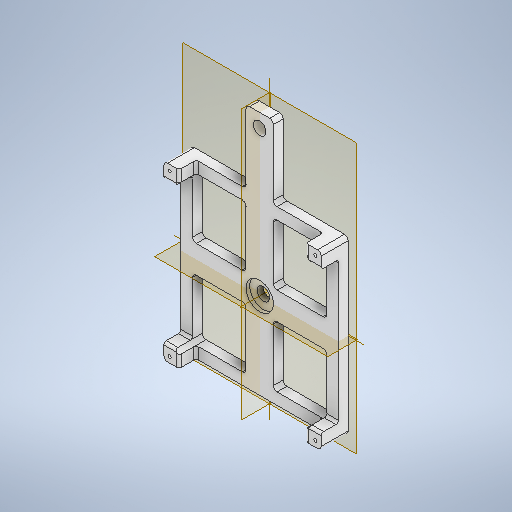
# Autodesk Inventor part: box-mount
Saved by Autodesk Inventor 2025.2 (Build 292293000, 293)
## iProperties
Created: 2025-04-08
Part Number: box-mount
Material: ABS Plastic
Document SubType Name: Modeling
Designer: yehorderehus
Density: 1.06 g/cm^3
Appearance: Smooth - White
Author: yehorderehus
Autodesk Inventor part; units mm, degrees
sketch "Sketch1" plane through (0, 0, 0) normal (0, 0, 1) x (1, 0, 0)
  line L0 (64.25, -70.25) -> (-64.25, -70.25)
  line L1 (-64.25, -70.25) -> (-64.25, 70.25)
  line L2 (-64.25, 70.25) -> (64.25, 70.25)
  line L3 (64.25, 70.25) -> (64.25, -70.25)
  circle A0 centre (0, 0) radius 5.2
  circle A1 centre (-59.5, -65.5) radius 1.25
  circle A2 centre (59.5, -65.5) radius 1.25
  circle A3 centre (59.5, 65.5) radius 1.25
  circle A4 centre (-59.5, 65.5) radius 1.25
  line L4 (-11.2, 70.25) -> (11.2, 70.25)
  line L5 (11.2, 70.25) -> (11.2, 129.75)
  line L6 (11.2, 129.75) -> (-11.2, 129.75)
  line L7 (-11.2, 129.75) -> (-11.2, 70.25)
  line L8 (0, 169.75) -> (0, -110.25) projected
  circle A5 centre (0, 118.55) radius 5.2
  line L9 (-54.75, 60.75) -> (-11.2, 60.75)
  line L10 (-11.2, 60.75) -> (-11.2, 11.2)
  line L11 (-11.2, 11.2) -> (-54.75, 11.2)
  line L12 (-54.75, 11.2) -> (-54.75, 60.75)
  line L13 (11.2, 11.2) -> (54.75, 11.2)
  line L14 (54.75, 11.2) -> (54.75, 60.75)
  line L15 (54.75, 60.75) -> (11.2, 60.75)
  line L16 (11.2, 60.75) -> (11.2, 11.2)
  line L17 (-11.2, -11.2) -> (-54.75, -11.2)
  line L18 (-54.75, -11.2) -> (-54.75, -60.75)
  line L19 (-54.75, -60.75) -> (-11.2, -60.75)
  line L20 (-11.2, -60.75) -> (-11.2, -11.2)
  line L21 (11.2, -11.2) -> (54.75, -11.2)
  line L22 (54.75, -11.2) -> (54.75, -60.75)
  line L23 (54.75, -60.75) -> (11.2, -60.75)
  line L24 (11.2, -60.75) -> (11.2, -11.2)
  line L25 (-89.95, 0) -> (89.95, 0) projected
  point P0 (11.2, 70.25)
  dimension "d0" = 10.4
  dimension "d12" = 119
  dimension "d14" = 131
  dimension "d44" = 3.5
  dimension "d45" = 3.5
  dimension "d46" = 3.5
  dimension "d47" = 3.5
  dimension "d48" = 3.5
  dimension "d49" = 3.5
  dimension "d50" = 6
  dimension "d51" = 6
  dimension "d52" = 3.5
  dimension "d53" = 65.5
  dimension "d54" = 2.5
  dimension "d55" = 59.5
  dimension "d56" = 6
  dimension "d57" = 3.5
  dimension "d58" = 6
  dimension "d60" = 6
  dimension "d62" = 200
  dimension "d63" = 118.55
  constraints: 48 end point, 12 equal length, 8 vertical alignment, 7 coincident, 6 centre point, 6 horizontal, 6 perpendicular, 4 equal radius, 4 horizontal alignment, 4 point on line
  measures "d0" diameter of A0
  measures "d12" distance of A1.centre A2.centre
  measures "d14" distance of A1.centre A4.centre
  measures "d44" distance edge to line of A1 L1
  measures "d45" distance edge to line of A1 L0
  measures "d46" distance edge to line of A4 L2
  measures "d47" distance edge to line of A2 L3
  measures "d48" distance edge to line of A1 L18
  measures "d49" distance edge to line of A2 L22
  measures "d50" distance edge to line of A0 L20
  measures "d51" distance edge to line of A0 L24
  measures "d52" distance edge to line of A1 L19
  measures "d53" distance from line of A1.centre L25
  measures "d54" diameter of A1
  measures "d55" distance from line of A1.centre L8
  measures "d56" distance edge to line of A0 L17
  measures "d57" distance edge to line of A4 L9
  measures "d58" distance edge to line of A0 L11
  measures "d60" distance edge to line of A5 L6
  measures "d62" distance between parallel lines of L0 L6
  measures "d63" distance of A0.centre A5.centre
extrude "Extrusion1" add sketch "Sketch1" along normal blind 8 contours L0 L8 A0 L25 L3 | L0 L1 L25 A0 L8 | L25 A0 L8 L2 L3 | L8 L25 A0 | A0 L25 L8 | L25 L8 A0 | L1 L2 L8 A0 L25 | A0 L8 L25 | L2 L8 A5 L6 L5 | L2 L7 L6 L8 A5 | A5 L8 | L8 A5 | A1 | A2 | A3 | A4
fillet "Fillet1" radius 3 24 edges at (64.25, 70.25, 4) (-64.25, 70.25, 4) (64.25, -70.25, 4) (-64.25, -70.25, 4) (11.2, 129.75, 4) (-11.2, 129.75, 4) (11.2, 70.25, 4) (-11.2, 70.25, 4) (-54.75, 60.75, 4) (-11.2, 60.75, 4) (-11.2, 11.2, 4) (-54.75, 11.2, 4) (11.2, 60.75, 4) (54.75, 60.75, 4) (11.2, 11.2, 4) (54.75, 11.2, 4) (-11.2, -11.2, 4) (-54.75, -11.2, 4) (-11.2, -60.75, 4) (-54.75, -60.75, 4) (11.2, -60.75, 4) (11.2, -11.2, 4) (54.75, -11.2, 4) (54.75, -60.75, 4)
hole "Hole1" at (59.5, 65.5, 0) at (-59.5, 65.5, 0) at (-59.5, -65.5, 0) at (59.5, -65.5, 0) direction (0, 0, 1) diameter 2.5 depth 8 counterbore diameter 6.4 counterbore depth 2
sketch "Sketch2" plane through (0, 0, 8) normal (0, 0, 1) x (1, 0, 0)
  line L0 (-89.95, 0) -> (89.95, 0) projected
  line L1 (0, 169.75) -> (0, -110.25) projected
  point P0 (0, 0)
  point P1 (0, 0)
  point P2 (0, 118.55)
  dimension "d71" = 118.55
  constraints: 1 coincident, 1 point on line
  measures "d71" distance from line of L0 point (0, 118.55)
hole "Hole2" at (0, 0, 8) direction (0, 0, -1) diameter 10.4 depth 8 counterbore diameter 22.4 counterbore depth 3
hole "Hole3" at (0, 118.55, 8) direction (0, 0, -1) diameter 10.4 depth 8
sketch "Sketch3" plane through (0, 0, 8) normal (0, 0, 1) x (1, 0, 0)
  circle A0 centre (-59.5, 65.5) radius 1.25 projected
  circle A1 centre (59.5, 65.5) radius 1.25 projected
  circle A2 centre (59.5, -65.5) radius 1.25 projected
  circle A3 centre (-59.5, -65.5) radius 1.25 projected
  arc A4 (-54.75, -57.75) -> (-51.75, -60.75) centre (-51.75, -57.75) ccw projected
  arc A5 (-51.75, 60.75) -> (-54.75, 57.75) centre (-51.75, 57.75) ccw projected
  arc A6 (54.75, 57.75) -> (51.75, 60.75) centre (51.75, 57.75) ccw projected
  arc A7 (64.25, 67.25) -> (61.25, 70.25) centre (61.25, 67.25) ccw projected
  arc A8 (-61.25, 70.25) -> (-64.25, 67.25) centre (-61.25, 67.25) ccw projected
  arc A9 (-64.25, -67.25) -> (-61.25, -70.25) centre (-61.25, -67.25) ccw projected
  arc A10 (61.25, -70.25) -> (64.25, -67.25) centre (61.25, -67.25) ccw projected
  arc A11 (51.75, -60.75) -> (54.75, -57.75) centre (51.75, -57.75) ccw projected
  line L0 (-14.2, 70.25) -> (-61.25, 70.25) projected
  line L1 (-51.75, 70.25) -> (-51.75, 60.75)
  line L2 (-64.25, 67.25) -> (-64.25, -67.25) projected
  line L3 (-64.25, 57.75) -> (-54.75, 57.75)
  line L4 (-64.25, -57.75) -> (-54.75, -57.75)
  line L5 (-51.75, -70.25) -> (-51.75, -60.75)
  line L6 (-61.25, -70.25) -> (61.25, -70.25) projected
  line L7 (51.75, -70.25) -> (51.75, -60.75)
  line L8 (64.25, -57.75) -> (54.75, -57.75)
  line L9 (51.75, 70.25) -> (51.75, 60.75)
  line L10 (64.25, -67.25) -> (64.25, 67.25) projected
  line L11 (64.25, 57.75) -> (54.75, 57.75)
  line L12 (61.25, 70.25) -> (14.2, 70.25) projected
  point P0 (0, 0)
  constraints: 16 end point, 7 perpendicular, 7 point on line, 1 horizontal
extrude "Extrusion2" add sketch "Sketch3" along normal blind 14
fillet "Fillet2" radius 2 16 edges at (-51.75, 65.5, 22) (-59.5, 57.75, 22) (51.75, 65.5, 22) (59.5, 57.75, 22) (-59.5, -57.75, 22) (-51.75, -65.5, 22) (51.75, -65.5, 22) (59.5, -57.75, 22) (-51.75, 65.5, 8) (-59.5, 57.75, 8) (51.75, 65.5, 8) (59.5, 57.75, 8) (59.5, -57.75, 8) (51.75, -65.5, 8) (-51.75, -65.5, 8) (-59.5, -57.75, 8)
equation "\"d46\" = d45"
equation "\"d47\" = d44"
equation "\"d48\" = d44"
equation "\"d49\" = d44"
equation "\"d52\" = d45"
equation "\"d53\" = 0.5 * d14"
equation "\"d55\" = 0.5 * d12"
body "Solid1"
